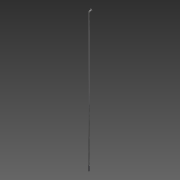
# Autodesk Inventor part: Szprycha
Saved by Autodesk Inventor 2015 (Build 190159000, 159)
## iProperties
Created: 2015-11-24
Part Number: Szprycha
Material: Stal nierdzewna
Document SubType Name: Modeling
Designer: graaapsik
Density: 8.08 g/cm^3
Appearance: Częściowo polerowany
Mass: 7.22889 g
Surface Area: 17.9054 cm^2
Volume: 0.894664 cm^3
Author: graaapsik
Autodesk Inventor part; units mm, degrees
ref_plane "YZ Plane" through (0, 0, 0) normal (1, 0, 0) x (0, 1, 0)
ref_plane "XZ Plane" through (0, 0, 0) normal (0, 1, 0) x (-1, 0, 0)
ref_plane "XY Plane" through (0, 0, 0) normal (0, 0, 1) x (1, 0, 0)
sketch "Szkic1" plane through (0, 0, 0) normal (0, 0, 1) x (1, 0, 0)
  circle A0 centre (0, 0) radius 1
  dimension "d0" = 2
  constraints: 1 centre point, 1 coincident
  measures "d0" diameter of A0
sketch "Szkic4" plane through (0, 0, 0) normal (1, 0, 0) x (0, 1, 0)
  line L0 (0, 0) -> (0, 263.8767)
  arc A0 (1.817, 265.8683) -> (0, 263.8767) centre (2, 263.8767) ccw
  line L1 (1.817, 265.8683) -> (3.25, 266)
  dimension "d2" = 266
  dimension "d3" = 2
  dimension "d4" = 3.25
  dimension "d5" = 95.25
  constraints: 4 end point, 2 point on circle, 2 tangent, 1 centre point, 1 vertical
  measures "d2" vertical distance of L0.start L1.end
  measures "d3" radius of A0
  measures "d4" distance from line of L1.end L0
  measures "d5" angle of L0 L1
sweep "Szprycha" add profiles "Szkic1" path "Szkic4"
sketch "Szkic5" plane through (0, 0, 0) normal (1, 0, 0) x (0, 1, 0)
  line L0 (3.3415, 265.0042) -> (3.1585, 266.9958) construction
  line L1 (3.1585, 266.9958) -> (3.25, 266)
  line L2 (3.1585, 266.9958) -> (4.1585, 268.1378)
  arc A0 (4.75, 266.1378) -> (4.1585, 268.1378) centre (-0.5843, 265.6477) ccw
  line L3 (1.7255, 266.8641) -> (3.1585, 266.9958) construction
  line L4 (1.9085, 264.8725) -> (3.3415, 265.0042) construction
  line L5 (1.9085, 264.8725) -> (1.7255, 266.8641) construction
  line L6 (1.817, 265.8683) -> (3.25, 266) construction
  line L7 (3.25, 266) -> (4.75, 266.1378)
  point P0 (0, 0)
  dimension "d7" = 1
  dimension "d8" = 1.5
  dimension "d10" = 2
  constraints: 8 end point, 2 midpoint, 2 point on circle, 1 centre point, 1 collinear, 1 line through centre, 1 perpendicular
  measures "d7" horizontal distance of L2.end L0.end
  measures "d8" horizontal distance of L1.end L7.end
  measures "d10" vertical distance of L7.end L2.end
revolve "Główka" add sketch "Szkic5" angle 360 about axis through (0, 3.25, 266) along (0, 0.9958049, 0.0915016)
sketch "Szkic6" plane through (0, 0, 0) normal (0, 0, 1) x (1, 0, 0)
  circle A0 centre (0, 0) radius 1.125
  dimension "d13" = 2.25
  constraints: 1 centre point, 1 coincident
  measures "d13" diameter of A0
extrude "Połączenie z nyplem" add sketch "Szkic6" against normal blind 10.3
chamfer "Faza1" distance 0.2 angle 45 1 edges at (-1.125, 0, -10.3)
thread "Gwint2"
